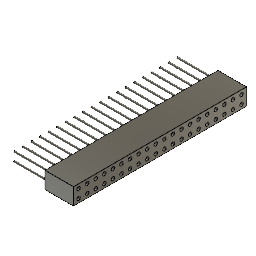
56b91e30-9c9f-4622-ba18-10aca97f1285 (Autodesk Fusion 360 design; units mm, degrees)
Autodesk Fusion 360 part; units mm, degrees
sketch "Sketch2" plane through (0, 0, 0) normal (1, 0, 0) x (0, 1, 0)
  line L0 (-58.52, 27.5) -> (-7.22, 27.5)
  line L1 (-7.22, 27.5) -> (-7.22, 22.5)
  line L2 (-7.22, 22.5) -> (-58.52, 22.5)
  line L3 (-58.52, 22.5) -> (-58.52, 27.5)
  circle A0 centre (-57, 23.73) radius 0.51
  circle A1 centre (-54.46, 23.73) radius 0.51
  circle A2 centre (-51.92, 23.73) radius 0.51
  circle A3 centre (-49.38, 23.73) radius 0.51
  circle A4 centre (-46.84, 23.73) radius 0.51
  circle A5 centre (-44.3, 23.73) radius 0.51
  circle A6 centre (-41.76, 23.73) radius 0.51
  circle A7 centre (-39.22, 23.73) radius 0.51
  circle A8 centre (-36.68, 23.73) radius 0.51
  circle A9 centre (-34.14, 23.73) radius 0.51
  circle A10 centre (-31.6, 23.73) radius 0.51
  circle A11 centre (-29.06, 23.73) radius 0.51
  circle A12 centre (-26.52, 23.73) radius 0.51
  circle A13 centre (-23.98, 23.73) radius 0.51
  circle A14 centre (-21.44, 23.73) radius 0.51
  circle A15 centre (-18.9, 23.73) radius 0.51
  circle A16 centre (-16.36, 23.73) radius 0.51
  circle A17 centre (-13.82, 23.73) radius 0.51
  circle A18 centre (-11.28, 23.73) radius 0.51
  circle A19 centre (-8.74, 23.73) radius 0.51
  circle A20 centre (-57, 26.27) radius 0.51
  circle A21 centre (-54.46, 26.27) radius 0.51
  circle A22 centre (-51.92, 26.27) radius 0.51
  circle A23 centre (-49.38, 26.27) radius 0.51
  circle A24 centre (-46.84, 26.27) radius 0.51
  circle A25 centre (-44.3, 26.27) radius 0.51
  circle A26 centre (-41.76, 26.27) radius 0.51
  circle A27 centre (-39.22, 26.27) radius 0.51
  circle A28 centre (-36.68, 26.27) radius 0.51
  circle A29 centre (-34.14, 26.27) radius 0.51
  circle A30 centre (-31.6, 26.27) radius 0.51
  circle A31 centre (-29.06, 26.27) radius 0.51
  circle A32 centre (-26.52, 26.27) radius 0.51
  circle A33 centre (-23.98, 26.27) radius 0.51
  circle A34 centre (-21.44, 26.27) radius 0.51
  circle A35 centre (-18.9, 26.27) radius 0.51
  circle A36 centre (-16.36, 26.27) radius 0.51
  circle A37 centre (-13.82, 26.27) radius 0.51
  circle A38 centre (-11.28, 26.27) radius 0.51
  circle A39 centre (-8.74, 26.27) radius 0.51
  line L4 (-57, 26.27) -> (-57, 23.73) construction
  line L5 (-57, 23.73) -> (-57, 25) construction
  line L6 (-57, 25) -> (-58.52, 25) construction
  line L7 (-8.74, 26.27) -> (-8.74, 23.73) construction
  line L8 (-8.74, 25) -> (-7.22, 25) construction
  dimension "d7" = 51.3
  dimension "d8" = 5
  dimension "d9" = 1.02
  dimension "d12" = 2.54
  dimension "d13" = 2.54
  constraint horizontal L0
  constraint vertical L1
  constraint horizontal L2
  constraint vertical L3
  constraint coincident A20.centre L4.start
  constraint coincident A0.centre L4.end
  constraint midpoint L4 L5.end
  constraint perpendicular L4 L6
  constraint midpoint L3 L6.end
  constraint coincident A39.centre L7.start
  constraint coincident A19.centre L7.end
  constraint midpoint L7 L8.start
  constraint midpoint L1 L8.end
  constraint equal L6 L8
  measures "d7" distance of L0.start L0.end
  measures "d8" distance of L0.start L2.end
  measures "d9" diameter of A0
extrude "Extrude2" add sketch "Sketch2" along normal blind 8.5 makes body 1
sketch "Sketch4" plane through (0, 0, 0) normal (1, 0, 0) x (0, 1, 0)
  circle A0 centre (-57, 26.27) radius 0.51
  circle A1 centre (-57, 26.27) radius 0.3
  circle A2 centre (-54.46, 26.27) radius 0.3
  circle A3 centre (-51.92, 26.27) radius 0.3
  circle A4 centre (-49.38, 26.27) radius 0.3
  circle A5 centre (-46.84, 26.27) radius 0.3
  circle A6 centre (-44.3, 26.27) radius 0.3
  circle A7 centre (-41.76, 26.27) radius 0.3
  circle A8 centre (-39.22, 26.27) radius 0.3
  circle A9 centre (-36.68, 26.27) radius 0.3
  circle A10 centre (-34.14, 26.27) radius 0.3
  circle A11 centre (-31.6, 26.27) radius 0.3
  circle A12 centre (-29.06, 26.27) radius 0.3
  circle A13 centre (-26.52, 26.27) radius 0.3
  circle A14 centre (-23.98, 26.27) radius 0.3
  circle A15 centre (-21.44, 26.27) radius 0.3
  circle A16 centre (-18.9, 26.27) radius 0.3
  circle A17 centre (-16.36, 26.27) radius 0.3
  circle A18 centre (-13.82, 26.27) radius 0.3
  circle A19 centre (-11.28, 26.27) radius 0.3
  circle A20 centre (-8.74, 26.27) radius 0.3
  circle A21 centre (-57, 23.73) radius 0.3
  circle A22 centre (-54.46, 23.73) radius 0.3
  circle A23 centre (-51.92, 23.73) radius 0.3
  circle A24 centre (-49.38, 23.73) radius 0.3
  circle A25 centre (-46.84, 23.73) radius 0.3
  circle A26 centre (-44.3, 23.73) radius 0.3
  circle A27 centre (-41.76, 23.73) radius 0.3
  circle A28 centre (-39.22, 23.73) radius 0.3
  circle A29 centre (-36.68, 23.73) radius 0.3
  circle A30 centre (-34.14, 23.73) radius 0.3
  circle A31 centre (-31.6, 23.73) radius 0.3
  circle A32 centre (-29.06, 23.73) radius 0.3
  circle A33 centre (-26.52, 23.73) radius 0.3
  circle A34 centre (-23.98, 23.73) radius 0.3
  circle A35 centre (-21.44, 23.73) radius 0.3
  circle A36 centre (-18.9, 23.73) radius 0.3
  circle A37 centre (-16.36, 23.73) radius 0.3
  circle A38 centre (-13.82, 23.73) radius 0.3
  circle A39 centre (-11.28, 23.73) radius 0.3
  circle A40 centre (-8.74, 23.73) radius 0.3
  dimension "d16" = 0.6
  dimension "d19" = 2.54
  dimension "d20" = -2.54
  constraint concentric A0 A1
  measures "d16" diameter of A1
extrude "Extrude3" add sketch "Sketch4" against normal blind 10.5 separate body contours A1 | A2 | A3 | A4 | A5 | A6 | A7 | A8 | A9 | A10 | A11 | A12 | A13 | A14 | A15 | A16 | A17 | A18 | A19 | A20 | A21 | A22 | A23 | A24 | A25 | A26 | A27 | A28 | A29 | A30 | A31 | A32 | A33 | A34 | A35 | A36 | A37 | A38 | A39 | A40 makes body 2 at (-7, -36.6875, 24.0299) makes body 3 at (-7, -34.1475, 26.5699) makes body 4 at (-7, -44.3075, 26.5699) makes body 5 at (-7, -29.3235, 26.1265) makes body 6 at (-7, -44.3075, 24.0299) makes body 7 at (-7, -11.5435, 26.1265) makes body 8 at (-7, -14.0835, 23.5865) makes body 9 at (-7, -21.7035, 26.1265) makes body 10 at (-7, -51.9275, 24.0299) makes body 11 at (-7, -57.0075, 24.0299) makes body 12 at (-7, -54.4675, 26.5699) makes body 13 at (-7, -9.0035, 26.1265) makes body 14 at (-7, -19.1635, 26.1265) makes body 15 at (-7, -24.2435, 23.5865) makes body 16 at (-7, -11.5435, 23.5865) makes body 17 at (-7, -39.2275, 24.0299) makes body 18 at (-7, -31.8635, 23.5865) makes body 19 at (-7, -39.2275, 26.5699) makes body 20 at (-7, -29.3235, 23.5865) makes body 21 at (-7, -46.8475, 24.0299) makes body 22 at (-7, -34.1475, 24.0299) makes body 23 at (-7, -36.6875, 26.5699) makes body 24 at (-7, -26.7835, 23.5865) makes body 25 at (-7, -26.7835, 26.1265) makes body 26 at (-7, -41.7675, 24.0299) makes body 27 at (-7, -14.0835, 26.1265) makes body 28 at (-7, -16.6235, 26.1265) makes body 29 at (-7, -24.2435, 26.1265) makes body 30 at (-7, -51.9275, 26.5699) makes body 31 at (-7, -57.0075, 26.5699) makes body 32 at (-7, -54.4675, 24.0299) makes body 33 at (-7, -9.0035, 23.5865) makes body 34 at (-7, -16.6235, 23.5865) makes body 35 at (-7, -21.7035, 23.5865) makes body 36 at (-7, -19.1635, 23.5865) makes body 37 at (-7, -31.8635, 26.1265) makes body 38 at (-7, -41.7675, 26.5699) makes body 39 at (-7, -49.3875, 26.5699) makes body 40 at (-7, -46.8475, 26.5699) makes body 41 at (-7, -49.3875, 24.0299)
equation "d7 = ( 2.54 * 20 ) * 1 mm + 0.5 mm"
